# Autodesk Inventor part: untitled.brd_Outline
Saved by Autodesk Inventor 2013 (Build 170138000, 138)
## iProperties
Created: 2014-11-03
Part Number: untitled.brd_Outline
Material: Generic
Document SubType Name: Modeling
Designer: Jeramy
Density: 1 g/cm^3
Author: Jeramy
Autodesk Inventor part; units mm, degrees
ref_plane "YZ Plane" through (0, 0, 0) normal (1, 0, 0) x (0, 1, 0)
ref_plane "XZ Plane" through (0, 0, 0) normal (0, 1, 0) x (-1, 0, 0)
ref_plane "XY Plane" through (0, 0, 0) normal (0, 0, 1) x (1, 0, 0)
sketch "Sketch1" plane through (0, 0, 0) normal (0, 0, 1) x (1, 0, 0)
  line L0 (55.88, 74.93) -> (55.88, 15.875)
  line L1 (55.88, 15.875) -> (43.18, 15.875)
  line L2 (43.18, 15.875) -> (42.9853, 17.3542)
  line L3 (42.9853, 17.3542) -> (42.4143, 18.7325)
  line L4 (42.4143, 18.7325) -> (41.5061, 19.9161)
  line L5 (41.5061, 19.9161) -> (40.3225, 20.8243)
  line L6 (40.3225, 20.8243) -> (38.9442, 21.3953)
  line L7 (38.9442, 21.3953) -> (37.465, 21.59)
  line L8 (37.465, 21.59) -> (19.685, 21.59)
  line L9 (19.685, 21.59) -> (18.2058, 21.3953)
  line L10 (18.2058, 21.3953) -> (16.8275, 20.8243)
  line L11 (16.8275, 20.8243) -> (15.6439, 19.9161)
  line L12 (15.6439, 19.9161) -> (14.7357, 18.7325)
  line L13 (14.7357, 18.7325) -> (14.1647, 17.3542)
  line L14 (14.1647, 17.3542) -> (13.97, 15.875)
  line L15 (13.97, 15.875) -> (1.27, 15.875)
  line L16 (1.27, 15.875) -> (1.27, 74.93)
  line L17 (1.27, 74.93) -> (1.7027, 78.217)
  line L18 (1.7027, 78.217) -> (2.9715, 81.28)
  line L19 (2.9715, 81.28) -> (4.9897, 83.9103)
  line L20 (4.9897, 83.9103) -> (7.62, 85.9285)
  line L21 (7.62, 85.9285) -> (10.683, 87.1973)
  line L22 (10.683, 87.1973) -> (13.97, 87.63)
  line L23 (13.97, 87.63) -> (43.18, 87.63)
  line L24 (43.18, 87.63) -> (46.467, 87.1973)
  line L25 (46.467, 87.1973) -> (49.53, 85.9285)
  line L26 (49.53, 85.9285) -> (52.1603, 83.9103)
  line L27 (52.1603, 83.9103) -> (54.1785, 81.28)
  line L28 (54.1785, 81.28) -> (55.4473, 78.217)
  line L29 (55.4473, 78.217) -> (55.88, 74.93)
  circle A0 centre (11.43, 81.28) radius 0.51
  circle A1 centre (13.97, 81.28) radius 0.51
  circle A2 centre (19.05, 81.28) radius 0.51
  circle A3 centre (21.59, 81.28) radius 0.51
  circle A4 centre (24.13, 81.28) radius 0.51
  circle A5 centre (26.67, 81.28) radius 0.51
  constraints: 60 end point, 6 centre point
extrude "untitled.brd_Outline" add sketch "Sketch1" along normal blind 1.6
body "Solid1"
